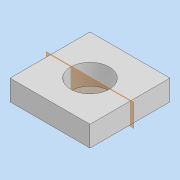
# Autodesk Inventor part: bearing2b
Saved by Autodesk Inventor 2022 (Build 260153000, 153)
## iProperties
Created: 2024-01-11
Part Number: bearing2b
Material: 一般
Document SubType Name: Modeling
Designer: ktamu
Density: 1 g/cm^3
Appearance: 既定
Author: ktamu
Autodesk Inventor part; units mm, degrees
ref_plane "YZ Plane" through (0, 0, 0) normal (1, 0, 0) x (0, 1, 0)
ref_plane "XZ Plane" through (0, 0, 0) normal (0, 1, 0) x (-1, 0, 0)
sketch "スケッチ1" plane through (0, 0, 0) normal (0, 1, 0) x (-1, 0, 0)
  circle A0 centre (0, 0) radius 15
  line L0 (31, 31) -> (-31, 31)
  line L1 (-31, 31) -> (-31, -31)
  line L2 (-31, -31) -> (31, -31)
  line L3 (31, -31) -> (31, 31)
  line L4 (31, 31) -> (-31, -31) construction
  line L5 (-31, 31) -> (31, -31) construction
  dimension "d0" = 30
  dimension "d1" = 62
  dimension "d2" = 62
  constraints: 12 end point, 2 midpoint, 2 parallel, 1 centre point, 1 coincident, 1 horizontal, 1 perpendicular
  measures "d0" diameter of A0
  measures "d1" distance of L2.end L1.end
  measures "d2" distance of L1.end L0.end
extrude "押し出し1" add sketch "スケッチ1" along normal blind 16
